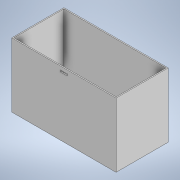
# Autodesk Inventor part: sciany boczne
Saved by Autodesk Inventor 2020.3 (Build 243373000, 373)
## iProperties
Created: 2021-01-13
Part Number: sciany boczne
Material: Ogólny
Document SubType Name: Modeling
Designer: sitar
Density: 1 g/cm^3
Appearance: Domyślna
Author: sitar
Autodesk Inventor part; units mm, degrees
ref_plane "YZ Plane" through (0, 0, 0) normal (1, 0, 0) x (0, 1, 0)
ref_plane "XZ Plane" through (0, 0, 0) normal (0, 1, 0) x (-1, 0, 0)
ref_plane "XY Plane" through (0, 0, 0) normal (0, 0, 1) x (1, 0, 0)
sketch "Szkic1" plane through (0, 0, 0) normal (0, 1, 0) x (-1, 0, 0)
  point P0 (0, 0)
sketch "Szkic2" plane through (0, 0, 0) normal (0, 1, 0) x (-1, 0, 0)
  line L0 (58.8, -28.8) -> (-58.8, -28.8)
  line L1 (-58.8, -28.8) -> (-58.8, 28.8)
  line L2 (-58.8, 28.8) -> (58.8, 28.8)
  line L3 (58.8, 28.8) -> (58.8, -28.8)
  line L4 (58.8, -28.8) -> (-58.8, 28.8) construction
  line L5 (-58.8, -28.8) -> (58.8, 28.8) construction
  line L6 (60, -30) -> (-60, -30)
  line L7 (-60, -30) -> (-60, 30)
  line L8 (-60, 30) -> (60, 30)
  line L9 (60, 30) -> (60, -30)
  line L10 (60, -30) -> (-60, 30) construction
  line L11 (-60, -30) -> (60, 30) construction
  line L12 (58.8, 28.8) -> (58.8, 30)
  point P0 (0, 0)
  dimension "d0" = 117.6
  dimension "d1" = 57.6
  dimension "d2" = 120
  dimension "d3" = 60
  constraints: 26 end point, 4 midpoint, 4 parallel, 2 horizontal, 2 perpendicular, 2 point on line
  measures "d0" distance of L1.end L2.end
  measures "d1" distance of L0.end L1.end
  measures "d2" distance of L7.end L8.end
  measures "d3" distance of L6.end L7.end
extrude "Wyciągnięcie proste1" add sketch "Szkic2" along normal blind 4
sketch "Szkic4" plane through (0, 4, 0) normal (0, 1, 0) x (1, 0, 0)
  line L0 (-60, 30) -> (60, 30)
  line L1 (60, 30) -> (60, -30)
  line L2 (60, -30) -> (-60, -30)
  line L3 (-60, -30) -> (-60, 30)
  line L4 (-60, 30) -> (60, -30) construction
  line L5 (60, 30) -> (-60, -30) construction
  line L6 (-57.6, 27.6) -> (57.6, 27.6)
  line L7 (57.6, 27.6) -> (57.6, -27.6)
  line L8 (57.6, -27.6) -> (-57.6, -27.6)
  line L9 (-57.6, -27.6) -> (-57.6, 27.6)
  line L10 (-57.6, 27.6) -> (57.6, -27.6) construction
  line L11 (57.6, 27.6) -> (-57.6, -27.6) construction
  line L12 (-57.6, 27.6) -> (-57.6, 30)
  point P0 (0, 0)
  dimension "d10" = 120
  dimension "d11" = 60
  dimension "d12" = 115.2
  dimension "d13" = 55.2
  constraints: 26 end point, 4 midpoint, 4 parallel, 3 perpendicular, 2 horizontal, 1 point on line
  measures "d10" distance of L1.end L2.end
  measures "d11" distance of L0.end L1.end
  measures "d12" distance of L7.end L8.end
  measures "d13" distance of L6.end L7.end
extrude "Wyciągnięcie proste2" add sketch "Szkic4" along normal blind 4
sketch "Szkic5" plane through (0, 8, 0) normal (0, 1, 0) x (1, 0, 0)
  line L0 (-58.8, 28.8) -> (58.8, 28.8)
  line L1 (58.8, 28.8) -> (58.8, -28.8)
  line L2 (58.8, -28.8) -> (-58.8, -28.8)
  line L3 (-58.8, -28.8) -> (-58.8, 28.8)
  line L4 (-58.8, 28.8) -> (58.8, -28.8) construction
  line L5 (58.8, 28.8) -> (-58.8, -28.8) construction
  line L6 (-60, 30) -> (60, 30)
  line L7 (60, 30) -> (60, -30)
  line L8 (60, -30) -> (-60, -30)
  line L9 (-60, -30) -> (-60, 30)
  line L10 (-60, 30) -> (60, -30) construction
  line L11 (60, 30) -> (-60, -30) construction
  line L12 (-58.8, 28.8) -> (58.8, 28.8) projected
  line L13 (-58.8, 28.8) -> (-58.8, 30)
  line L14 (60, 30) -> (-60, 30) projected
  point P0 (0, 0)
  dimension "d16" = 117.6
  dimension "d17" = 57.6
  dimension "d18" = 120
  dimension "d19" = 60
  constraints: 26 end point, 4 midpoint, 4 parallel, 2 horizontal, 2 perpendicular, 1 point on line, 1 vertical
  measures "d16" distance of L1.end L2.end
  measures "d17" distance of L0.end L1.end
  measures "d18" distance of L7.end L8.end
  measures "d19" distance of L6.end L7.end
extrude "Wyciągnięcie proste3" add sketch "Szkic5" along normal blind 66
sketch "Szkic8" plane through (0, 4, 0) normal (0, -1, 0) x (1, 0, 0)
  line L0 (57.6, -28.8) -> (-57.6, -28.8)
  line L1 (-57.6, -28.8) -> (-57.6, 28.8)
  line L2 (-57.6, 28.8) -> (57.6, 28.8)
  line L3 (57.6, 28.8) -> (57.6, -28.8)
  line L4 (57.6, -28.8) -> (-57.6, 28.8) construction
  line L5 (-57.6, -28.8) -> (57.6, 28.8) construction
  point P0 (0, 0)
  dimension "d30" = 115.2
  dimension "d31" = 57.6
  constraints: 12 end point, 2 midpoint, 2 parallel, 1 horizontal, 1 perpendicular
  measures "d30" distance of L1.end L2.end
  measures "d31" distance of L0.end L1.end
extrude "Wyciągnięcie proste5" cut sketch "Szkic8" against normal through all
sketch "Szkic9" plane through (-60, 0, 30) normal (0, 0, 1) x (1, 0, 0)
  line L0 (60, 0) -> (60, 69)
  line L1 (60, 0) -> (129, 0) construction
  line L2 (64, 68) -> (56, 68)
  line L3 (56, 68) -> (56, 70)
  line L4 (56, 70) -> (64, 70)
  line L5 (64, 70) -> (64, 68)
  line L6 (64, 68) -> (56, 70) construction
  line L7 (56, 68) -> (64, 70) construction
  dimension "d34" = 69
  dimension "d35" = 90
  dimension "d36" = 8
  dimension "d37" = 2
  constraints: 16 end point, 2 horizontal, 2 midpoint, 2 parallel, 2 perpendicular, 1 vertical
  measures "d34" distance of L0.start L0.end
  measures "d35" angle of L1 L0
  measures "d36" distance of L3.end L4.end
  measures "d37" distance of L2.end L3.end
extrude "Wyciągnięcie proste6" cut sketch "Szkic9" against normal blind 10
